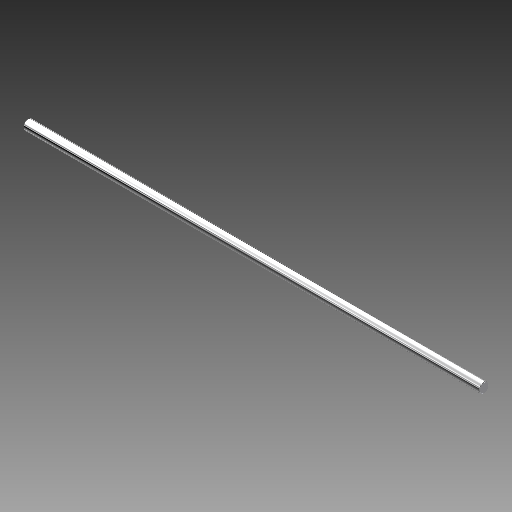
# Autodesk Inventor part: Eje Principal - Interno
Saved by Autodesk Inventor 2019 (Build 230136000, 136)
## iProperties
Created: 2019-09-30
Part Number: Eje Principal - Interno
Material: Aluminum 6061
Document SubType Name: Modeling
Designer: Domenico
Density: 2.7 g/cm^3
Appearance: Aluminum - Flat
Mass: 629.256 g
Surface Area: 376.632 cm^2
Volume: 233.058 cm^3
CustomPartVersion: 1
Author: Domenico
Autodesk Inventor part; units mm, degrees
ref_plane "Start Plane" through (0, 0, 0) normal (1, 0, 0) x (0, 1, 0)
ref_plane "XZ Plane" through (0, 0, 0) normal (0, 1, 0) x (-1, 0, 0)
ref_plane "XY Plane" through (0, 0, 0) normal (0, 0, 1) x (1, 0, 0)
sketch "Main Sketch" plane through (0, 0, 0) normal (0, 0, 1) x (1, 0, 0)
  line L0 (0, 0) -> (460, 0)
  line L1 (460, 5) -> (460, 0)
  line L2 (10, 5) -> (460, 5)
  line L3 (0, 0) -> (0, 5)
  line L4 (0, 5) -> (10, 5)
  dimension "d3" = 10
  dimension "d15" = 10
  constraints: 10 end point, 2 horizontal, 2 vertical
  measures "d3" diameter of L2 L0
  measures "d15" diameter of L4 L0
revolve "Revolution1" add sketch "Main Sketch" angle 360 about axis through (0, 0, 0) along (1, 0, 0)
chamfer "Chamfer4" distance 0.595 angle 45 1 edges at (0, -5, 0) measured on face at (3.3333, 4.9353, -0.8021)
chamfer "Chamfer3" distance 0.595 angle 45 1 edges at (460, -5, 0) measured on face at (160, 4.9838, -0.4023)
body "Solid1"
